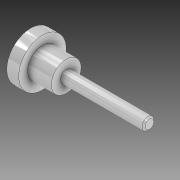
# Autodesk Inventor part: FE-120-008 Pin
Saved by Autodesk Inventor 2021 (Build 250183000, 183)
## iProperties
Created: 2021-01-12
Part Number: FE-120-008 Pin
Material: Aluminum 6061
Document SubType Name: Modeling
Density: 2.7 g/cm^3
Appearance: Aluminum - Dark
Autodesk Inventor part; units mm, degrees
ref_plane "YZ Plane" through (0, 0, 0) normal (1, 0, 0) x (0, 1, 0)
ref_plane "XZ Plane" through (0, 0, 0) normal (0, 1, 0) x (-1, 0, 0)
ref_plane "XY Plane" through (0, 0, 0) normal (0, 0, 1) x (1, 0, 0)
sketch "Sketch1" plane through (0, 0, 0) normal (0, 0, 1) x (1, 0, 0)
  line L0 (-31.75, 0) -> (31.75, 0)
  line L1 (-31.75, 0) -> (-31.75, 12.7)
  line L2 (-31.75, 12.7) -> (-25.4, 12.7)
  line L3 (-25.4, 12.7) -> (-25.4, 7.9375)
  line L4 (-25.4, 7.9375) -> (-12.7, 7.9375)
  line L5 (-12.7, 7.9375) -> (-12.7, 3.175)
  line L6 (-12.7, 3.175) -> (31.75, 3.175)
  line L7 (31.75, 3.175) -> (31.75, 0)
  point P0 (0, 0)
  point P1 (0, 0)
  dimension "d0" = 25.4
  dimension "d1" = 15.875
  dimension "d2" = 6.35
  dimension "d3" = 6.35
  dimension "d4" = 12.7
  dimension "d5" = 44.45
  constraints: 17 end point, 6 perpendicular, 1 coincident, 1 horizontal, 1 midpoint, 1 vertical
  measures "d0" diameter of L2 L0
  measures "d1" diameter of L4 L0
  measures "d2" diameter of L6 L0
  measures "d3" distance of L1.end L2.end
  measures "d4" distance of L3.end L4.end
  measures "d5" distance between parallel lines of L7 L5
revolve "Revolution1" add sketch "Sketch1" angle 360 about axis through (-31.75, 0, 0) along (1, 0, 0)
chamfer "Chamfer1" distance 0.7937 angle 45 1 edges at (31.75, -3.175, 0)
body "Solid1"
